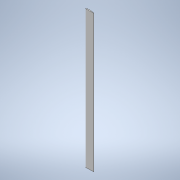
# Autodesk Inventor part: propeller mould
Saved by Autodesk Inventor 2022 (Build 260153000, 153)
## iProperties
Created: 2021-03-18
Part Number: propeller mould
Material: Generic
Document SubType Name: Modeling
Designer: Ferdinand Hubbard
Density: 1 g/cm^3
Appearance: Default
Author: Ferdinand Hubbard
Autodesk Inventor part; units mm, degrees
ref_plane "YZ Plane" through (0, 0, 0) normal (1, 0, 0) x (0, 1, 0)
ref_plane "XZ Plane" through (0, 0, 0) normal (0, 1, 0) x (-1, 0, 0)
ref_plane "XY Plane" through (0, 0, 0) normal (0, 0, 1) x (1, 0, 0)
sketch "Sketch1" plane through (0, 0, 0) normal (0, 1, 0) x (-1, 0, 0)
  spline S0 degree 4 poles (-20, -0.026) (-19.0708, -0.2726) (-18.7785, -0.3708) (-16.3038, -0.9518) (-14.0016, -1.3452) (-12.0127, -1.6501) (-9.9945, -1.8449) (-8.2771, -1.9864) (-6.0795, -1.9741) (-5.1588, -1.9078) (-3.9991, -1.7707) (-3.1236, -1.6222) (-2.043, -1.3459) (-1.5545, -1.1707) (-1.0588, -0.9994) (-0.4556, -0.6494) (-0.3069, -0.5813) (0.2019, 0.0183) (-0.2953, 0.3258) (-0.4703, 0.3919) (-1.0736, 0.5287) (-1.5612, 0.5489) (-2.0538, 0.585) (-3.1352, 0.5788) (-4.0054, 0.5528) (-5.163, 0.4897) (-6.0814, 0.4494) (-8.2744, 0.3427) (-9.9901, 0.2837) (-12.0046, 0.1963) (-13.9946, 0.1269) (-16.2883, 0.0656) (-18.7703, 0.0275) (-19.0701, 0.0421) (-20, 0) knots 0 0 0 0 0 0.079488 0.116387 0.156095 0.195698 0.235222 0.271815 0.305519 0.336384 0.364476 0.390648 0.414949 0.437473 0.456817 0.476263 0.494879 0.511872 0.529944 0.547796 0.566284 0.588116 0.611934 0.637786 0.665681 0.696468 0.730146 0.766712 0.806164 0.845613 0.885058 0.921612 1 1 1 1 1
  line L0 (-20, 0) -> (-20, -0.026)
  point P0 (0, 0)
  point P1 (-19, -0.294)
  point P2 (-18, -0.542)
  point P3 (-16, -0.978)
  point P4 (-14, -1.338)
  point P5 (-12, -1.628)
  point P6 (-10, -1.838)
  point P7 (-8, -1.96)
  point P8 (-6, -1.952)
  point P9 (-5, -1.882)
  point P10 (-4, -1.76)
  point P11 (-3, -1.578)
  point P12 (-2, -1.318)
  point P13 (-1.5, -1.152)
  point P14 (-1, -0.946)
  point P15 (-0.5, -0.678)
  point P16 (-0.25, -0.488)
  point P17 (0, 0)
  point P18 (-0.25, 0.286)
  point P19 (-0.5, 0.39)
  point P20 (-1, 0.498)
  point P21 (-1.5, 0.548)
  point P22 (-2, 0.572)
  point P23 (-3, 0.576)
  point P24 (-4, 0.548)
  point P25 (-5, 0.5)
  point P26 (-6, 0.452)
  point P27 (-8, 0.36)
  point P28 (-10, 0.28)
  point P29 (-12, 0.2)
  point P30 (-14, 0.13)
  point P31 (-16, 0.078)
  point P32 (-18, 0.044)
  point P33 (-19, 0.032)
  constraints: 2 end point, 1 vertical, 35 other
sketch "Sketch2" plane through (0, 0, 0) normal (0, 0, 1) x (1, 0, 0)
  line L0 (0, 0) -> (0, 330)
  dimension "d0" = 330
  constraints: 2 end point, 1 vertical
  measures "d0" distance of L0.start L0.end
sweep "Sweep1" add profiles "Sketch1" path "Sketch2"
body "Solid1"
